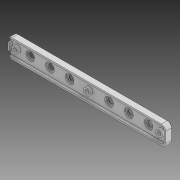
# Autodesk Inventor part: LEDHolder
Saved by Autodesk Inventor 2020 (Build 240168000, 168)
## iProperties
Created: 2020-12-20
Part Number: LEDHolder
Material: Generic
Document SubType Name: Modeling
Designer: DDeGo
Density: 1 g/cm^3
Appearance: Default
Author: DDeGo
Autodesk Inventor part; units mm, degrees
sketch "Sketch1" plane through (0, 0, 0) normal (0, 0, 1) x (1, 0, 0)
  line L0 (-75, -9) -> (75, -9)
  line L1 (75, -9) -> (75, 9)
  line L2 (75, 9) -> (-75, 9)
  line L3 (-75, 9) -> (-75, -9)
  line L4 (-75, -9) -> (75, 9) construction
  line L5 (75, -9) -> (-75, 9) construction
  point P0 (0, 0)
  dimension "d0" = 150
  dimension "d1" = 18
  constraints: 12 end point, 2 midpoint, 2 parallel, 1 horizontal, 1 perpendicular
  measures "d0" distance of L1.end L2.end
  measures "d1" distance of L0.end L1.end
extrude "Extrusion1" add sketch "Sketch1" along normal blind 3.5
sketch "Sketch2" plane through (0, 0, 3.5) normal (0, 0, 1) x (1, 0, 0)
  line L0 (0, 0) -> (-18.75, 0) construction
  line L1 (-18.75, 0) -> (-37.5, 0) construction
  line L2 (-37.5, 0) -> (-56.25, 0) construction
  line L3 (-56.25, 0) -> (-75, 0) construction
  line L4 (-75, 9) -> (-75, -9) construction
  line L5 (0, 0) -> (18.75, 0) construction
  line L6 (18.75, 0) -> (37.5, 0) construction
  line L7 (37.5, 0) -> (56.25, 0) construction
  line L8 (56.25, 0) -> (75, 0) construction
  line L9 (75, -9) -> (75, 9) construction
  dimension "d16" = 18.75
  constraints: 16 end point, 6 coincident, 6 collinear, 5 point on line, 2 midpoint, 1 horizontal
  measures "d16" distance of L1.end L2.end
ref_plane "Work Plane1" through (-56.25, 0, 3.5) normal (1, 0, 0) x (0, 1, 0)
sketch "Sketch3" plane through (-56.25, 0, 3.5) normal (1, 0, 0) x (0, 1, 0)
  line L0 (9, -3.5) -> (-9, -3.5) construction
  line L1 (0, 0) -> (-4.15, 0)
  line L2 (-4.15, 0) -> (-4.15, -1)
  line L3 (-4.15, -1) -> (-2.8, -1)
  arc A0 (-2.8, -1) -> (-2.6153, -2) centre (0, -1) ccw
  line L4 (0, 0) -> (0, -3.5)
  line L5 (-2.6153, -2) -> (-4.1153, -3.5)
  line L6 (-4.1153, -3.5) -> (0, -3.5)
  arc A1 (-2.6153, -2) -> (0, -3.8) centre (0, -1) ccw construction
  line L7 (-9, -3.5) -> (9, -3.5) projected
  line L8 (0, -3.5) -> (0, -3.8) construction
  dimension "d4" = 4.15
  dimension "d5" = 2.8
  dimension "d6" = 1
  dimension "d7" = 1
  dimension "d8" = 45
  constraints: 14 end point, 4 point on circle, 3 horizontal, 2 centre point, 2 midpoint, 2 point on line, 2 vertical, 1 collinear, 1 perpendicular
  measures "d4" distance of L1.start L1.end
  measures "d5" horizontal distance of L1.start L3.end
  measures "d6" distance of L1.end L2.end
  measures "d7" distance from line of L3 L5.start
  measures "d8" angle of L3 L5
revolve "Revolution1" cut sketch "Sketch3" angle 360 about axis through (-56.25, 0, 3.5) along (0, 0, -1)
sketch "Sketch4" plane through (0, 0, 3.5) normal (0, 0, 1) x (1, 0, 0)
  line L0 (-60.4, 1.1057) -> (-60.25, 1.1057)
  line L1 (-60.25, 1.1057) -> (-60.25, -1.1057)
  line L2 (-60.25, -1.1057) -> (-60.4, -1.1057)
  line L3 (-60.4, -1.1057) -> (-60.4, 1.1057)
  line L4 (-56.25, 0) -> (-56.25, 1.7802) construction
  circle A0 centre (-56.25, 0) radius 4.15 construction
  line L5 (-52.1, 1.1057) -> (-52.25, 1.1057)
  line L6 (-52.25, 1.1057) -> (-52.25, -1.1057)
  line L7 (-52.25, -1.1057) -> (-52.1, -1.1057)
  line L8 (-52.1, -1.1057) -> (-52.1, 1.1057)
  point P0 (0, 0)
  dimension "d10" = 4
  constraints: 18 end point, 4 symmetric about line, 2 parallel, 2 point on circle, 1 horizontal, 1 perpendicular, 1 tangent, 1 vertical
  measures "d10" distance between parallel lines of L4 L1
extrude "Extrusion2" add sketch "Sketch4" against normal up to surface (1 mm away)
pattern_linear "Rectangular Pattern1" count 3 spacing 18.75 along (1, 0, 0) of "Revolution1", "Extrusion2"
mirror "Mirror1" about plane through (0, 0, 0) normal (1, 0, 0) of "Revolution1", "Extrusion2", "Rectangular Pattern1"
fillet "Fillet1" radius 4 4 edges at (-75, -9, 1.75) (-75, 9, 1.75) (75, -9, 1.75) (75, 9, 1.75)
ref_plane "LED Backside" through (-56.25, 0, 6) normal (0, 0, 1) x (1, 0, 0)
sketch "Sketch5" plane through (0, 0, 3.5) normal (0, 0, 1) x (1, 0, 0)
  line L0 (22.75, -1.1057) -> (22.75, 1.1057) projected
  arc A0 (14.75, -1.1057) -> (22.75, -1.1057) centre (18.75, 0) ccw projected
  line L1 (14.75, 1.1057) -> (14.75, -1.1057) projected
  arc A1 (22.75, 1.1057) -> (14.75, 1.1057) centre (18.75, 0) ccw projected
  line L2 (41.5, -1.1057) -> (41.5, 1.1057) projected
  arc A2 (33.5, -1.1057) -> (41.5, -1.1057) centre (37.5, 0) ccw projected
  line L3 (33.5, 1.1057) -> (33.5, -1.1057) projected
  arc A3 (41.5, 1.1057) -> (33.5, 1.1057) centre (37.5, 0) ccw projected
  line L4 (-60.25, -1.1057) -> (-60.25, 1.1057) projected
  arc A4 (-52.25, 1.1057) -> (-60.25, 1.1057) centre (-56.25, 0) ccw projected
  line L5 (-52.25, 1.1057) -> (-52.25, -1.1057) projected
  arc A5 (-60.25, -1.1057) -> (-52.25, -1.1057) centre (-56.25, 0) ccw projected
  arc A6 (75, 5) -> (71, 9) centre (71, 5) ccw projected
  line L6 (71, 9) -> (-71, 9) projected
  arc A7 (-71, 9) -> (-75, 5) centre (-71, 5) ccw projected
  line L7 (-75, 5) -> (-75, -5) projected
  arc A8 (-75, -5) -> (-71, -9) centre (-71, -5) ccw projected
  line L8 (-71, -9) -> (71, -9) projected
  arc A9 (71, -9) -> (75, -5) centre (71, -5) ccw projected
  line L9 (75, -5) -> (75, 5) projected
  line L10 (-41.5, -1.1057) -> (-41.5, 1.1057) projected
  arc A10 (-33.5, 1.1057) -> (-41.5, 1.1057) centre (-37.5, 0) ccw projected
  line L11 (-33.5, 1.1057) -> (-33.5, -1.1057) projected
  arc A11 (-41.5, -1.1057) -> (-33.5, -1.1057) centre (-37.5, 0) ccw projected
  line L12 (-22.75, -1.1057) -> (-22.75, 1.1057) projected
  arc A12 (-14.75, 1.1057) -> (-22.75, 1.1057) centre (-18.75, 0) ccw projected
  line L13 (-14.75, 1.1057) -> (-14.75, -1.1057) projected
  arc A13 (-22.75, -1.1057) -> (-14.75, -1.1057) centre (-18.75, 0) ccw projected
  line L14 (60.25, -1.1057) -> (60.25, 1.1057) projected
  arc A14 (52.25, -1.1057) -> (60.25, -1.1057) centre (56.25, 0) ccw projected
  line L15 (52.25, 1.1057) -> (52.25, -1.1057) projected
  arc A15 (60.25, 1.1057) -> (52.25, 1.1057) centre (56.25, 0) ccw projected
  line L16 (-71, 7.5) -> (71, 7.5)
  arc A16 (73.5, 5) -> (71, 7.5) centre (71, 5) ccw
  line L17 (73.5, 5) -> (73.5, -5)
  arc A17 (71, -7.5) -> (73.5, -5) centre (71, -5) ccw
  line L18 (71, -7.5) -> (-71, -7.5)
  arc A18 (-73.5, -5) -> (-71, -7.5) centre (-71, -5) ccw
  line L19 (-73.5, -5) -> (-73.5, 5)
  arc A19 (-71, 7.5) -> (-73.5, 5) centre (-71, 5) ccw
  circle A20 centre (0, 0) radius 1.4
  circle A21 centre (-68.5, 0) radius 1.4
  circle A22 centre (68.5, 0) radius 1.4
  circle A23 centre (-68.5, 0) radius 3.25
  circle A24 centre (0, 0) radius 3.25
  circle A25 centre (68.5, 0) radius 3.25
  dimension "d19" = 1.5
  dimension "d21" = 12.25
  dimension "d22" = 12.25
  dimension "d23" = 2.8
  dimension "d24" = 6.5
  dimension "d33" = 6.5
  dimension "d34" = 5
  constraints: 10 centre point, 8 end point, 8 point on circle, 4 coincident, 4 equal radius, 2 horizontal alignment, 7 other
  measures "d19" distance between parallel lines of L6 L16
  measures "d21" distance of A4.centre A21.centre
  measures "d22" distance of A22.centre A14.centre
  measures "d23" diameter of A20
  measures "d24" diameter of A24
  measures "d33" distance from line of A21.centre L7
  measures "d34" distance from line of L17 A22.centre
extrude "Extrusion3" add sketch "Sketch5" along normal up to surface (2.5 mm away) contours L9 A9 L8 A8 L7 A7 L6 A6 | A23 | A24 | A25
ref_plane "Work Plane3" through (0, 0, 0.8) normal (0, 0, -1) x (-1, 0, 0)
sketch "Sketch6" plane through (-68.5, 0, 3.5) normal (0, 0, 1) x (1, 0, 0)
  circle A0 centre (0, 0) radius 1.4 projected
  circle A1 centre (68.5, 0) radius 1.4 projected
  circle A2 centre (137, 0) radius 1.4 projected
extrude "Extrusion4" cut sketch "Sketch6" against normal up to surface (2.7 mm away)
chamfer "Chamfer1" distance 0.5 angle 45 3 edges at (-69.9, 0, 6) (-1.4, 0, 6) (67.1, 0, 6)
sketch "Sketch7" plane through (-71, -9, 6) normal (0, 0, 1) x (1, 0, 0)
  line L0 (0, 1.5) -> (142, 1.5) projected
  line L1 (0, 1.5) -> (-6.2457, 1.5)
  line L2 (-6.2457, 1.5) -> (-6.2457, 5.5)
  line L3 (-6.2457, 5.5) -> (0, 5.5)
  line L4 (0, 5.5) -> (0, 1.5)
  line L5 (142, 16.5) -> (0, 16.5) projected
  line L6 (0, 16.5) -> (-6.2457, 16.5)
  line L7 (-6.2457, 16.5) -> (-6.2457, 12.5)
  line L8 (-6.2457, 12.5) -> (0, 12.5)
  line L9 (0, 12.5) -> (0, 16.5)
  point P0 (71, 9)
  dimension "d35" = 4
  constraints: 16 end point, 4 parallel, 2 horizontal, 2 perpendicular, 1 collinear
  measures "d35" distance of L3.end L0.start
extrude "Extrusion5" cut sketch "Sketch7" against normal up to surface (2.5 mm away)
chamfer "Chamfer2" distance 0.5 angle 45 8 edges at (0, 9, 0) (-73.8284, 7.8284, 0) (-75, 0, 0) (-73.8284, -7.8284, 0) (0, -9, 0) (73.8284, -7.8284, 0) (75, 0, 0) (73.8284, 7.8284, 0)
equation "\"d15\" = d16"
equation "\"d22\" = d21"
body "Solid1"
